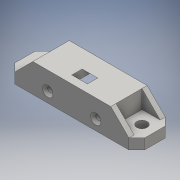
# Autodesk Inventor part: Support_GP2
Saved by Autodesk Inventor 2016 (Build 200138000, 138)
## iProperties
Created: 2016-09-29
Part Number: Support_GP2
Material: Générique
Document SubType Name: Modeling
Designer: LogOut
Density: 1 g/cm^3
Appearance: Par défaut
Author: LogOut
Autodesk Inventor part; units mm, degrees
ref_plane "YZ Plane" through (0, 0, 0) normal (1, 0, 0) x (0, 1, 0)
ref_plane "XZ Plane" through (0, 0, 0) normal (0, 1, 0) x (-1, 0, 0)
sketch "Esquisse1" plane through (0, 0, 0) normal (0, 0, 1) x (1, 0, 0)
  line L0 (-50, 14) -> (50, 14)
  line L1 (50, 14) -> (50, -14)
  line L2 (50, -14) -> (-50, -14)
  line L3 (-50, -14) -> (-50, 14)
  point P0 (0, 0)
  dimension "d0" = 100
  dimension "d1" = 28
  dimension "d2" = 14
  dimension "d3" = 50
  constraints: 8 end point, 2 parallel, 1 horizontal, 1 perpendicular
  measures "d0" distance of L0.start L0.end
  measures "d1" distance of L2.end L0.start
  measures "d2" distance from line of point (0, 0) L0
  measures "d3" distance from line of point (0, 0) L1
extrude "Extrusion1" add sketch "Esquisse1" along normal blind 28
sketch "Esquisse2" plane through (-50, 14, 0) normal (0, 1, 0) x (1, 0, 0)
  line L0 (26, -22) -> (74, -22)
  line L1 (74, -22) -> (74, -6)
  line L2 (74, -6) -> (26, -6)
  line L3 (26, -6) -> (26, -22)
  line L4 (0, 0) -> (100, 0) projected
  line L5 (0, 0) -> (0, -28) projected
  line L6 (100, -28) -> (0, -28) projected
  line L7 (100, 0) -> (100, -28) projected
  point P0 (50, 0)
  dimension "d6" = 26
  dimension "d7" = 48
  dimension "d8" = 26
  dimension "d9" = 6
  dimension "d10" = 6
  dimension "d11" = 16
  constraints: 8 end point, 2 parallel, 1 horizontal, 1 perpendicular
  measures "d6" distance between parallel lines of L5 L3
  measures "d7" distance between parallel lines of L1 L3
  measures "d8" distance between parallel lines of L7 L1
  measures "d9" distance between parallel lines of L4 L2
  measures "d10" distance between parallel lines of L6 L0
  measures "d11" distance of L2.end L0.start
extrude "Extrusion2" cut sketch "Esquisse2" against normal blind 24 contours L3 L2 L1 L0
ref_plane "Plan de construction1" through (-24, 14, 14) normal (0, 0, 1) x (1, 0, 0)
sketch "Esquisse3" plane through (-24, 14, 14) normal (0, 0, 1) x (1, 0, 0)
  line L0 (110.7171, 2) -> (-26, 2)
  line L1 (70, 2) -> (54, -18)
  line L2 (-6, -18) -> (-26, 2)
  line L3 (-26, 2) -> (-81.3521, 2)
  line L4 (74, -28) -> (-26, -28) projected
  line L5 (110.7171, 2) -> (110.7171, -53.3012)
  line L6 (110.7171, -53.3012) -> (-81.3521, -53.3012)
  line L7 (-81.3521, -53.3012) -> (-81.3521, 2)
  line L8 (-6, 2) -> (-6, -28)
  line L9 (-26, -28) -> (74, -28) projected
  line L10 (-6, -28) -> (54, -28)
  line L11 (54, -53.3012) -> (54, 2)
  point P0 (24, -14)
  point P1 (54.2399, -28)
  point P2 (-6.2399, -28)
  dimension "d25" = 60
  dimension "d26" = 30
  dimension "d27" = 30
  constraints: 20 end point, 10 point on line, 5 perpendicular, 1 collinear, 1 horizontal, 1 vertical
  measures "d25" distance between parallel lines of L11 L8
  measures "d26" distance from line of point (24, -14) L11
  measures "d27" distance from line of point (24, -14) L8
extrude "Extrusion3" cut sketch "Esquisse3" along normal blind 14 and the other way blind 3 contours L5 L6 L11 L1 L0 | L1 L11 L0 | L6 L7 L3 L2 L8 L4 L11 | L8 L2 L0
sketch "Esquisse7" plane through (-50, -10, 0) normal (0, 1, 0) x (1, 0, 0)
  line L0 (68.5, -14) -> (31.5, -14)
  line L1 (74, -6) -> (74, -22) projected
  line L2 (26, -6) -> (74, -6) projected
  point P0 (50, 0)
  dimension "d61" = 37
  dimension "d62" = 5.5
  dimension "d63" = 8
  constraints: 2 end point, 1 horizontal
  measures "d61" distance of L0.start L0.end
  measures "d62" distance from line of L1 L0.start
  measures "d63" distance between parallel lines of L0 L2
hole "Perçage2" at (18.5, -10, 14) at (-18.5, -10, 14) direction (0, -1, 0) diameter 4 end through all
chamfer "Chanfrein1" distance 2 angle 45 6 edges at (-18.5, -14, 12) (18.5, -14, 12) (24, 14, 14) (0, 14, 22) (-24, 14, 14) (0, 14, 6)
sketch "Esquisse8" plane through (0, 0, 28) normal (0, 0, 1) x (1, 0, 0)
  line L0 (6, -8) -> (-6, -8)
  line L1 (-6, -8) -> (-6, 0)
  line L2 (-6, 0) -> (6, 0)
  line L3 (6, 0) -> (6, -8)
  line L4 (-30, -14) -> (30, -14) projected
  point P0 (0, 0)
  point P1 (-28, -14)
  point P2 (28, -14)
  dimension "d74" = 12
  dimension "d75" = 8
  dimension "d76" = 6
  dimension "d77" = 6
  constraints: 8 end point, 2 parallel, 1 horizontal, 1 perpendicular
  measures "d74" distance of L0.start L0.end
  measures "d75" distance between parallel lines of L0 L2
  measures "d76" distance between parallel lines of L4 L0
  measures "d77" distance from line of point (0, 0) L3
extrude "Extrusion6" cut sketch "Esquisse8" against normal blind 6
chamfer "Chanfrein2" distance 8 distance2 6 1 edges at (0, 0, 22) measured on face at (2, 8, 22)
sketch "Esquisse10" plane through (-50, 14, 11) normal (0, 1, 0) x (1, 0, 0)
  line L0 (26, 5) -> (74, 5) projected
  line L1 (0, 11) -> (0, 0) projected
  line L2 (100, 11) -> (100, 0) projected
  line L3 (108, 0) -> (100, 0) projected
  line L4 (100, 0) -> (100, 29.3143)
  line L5 (100, 29.3143) -> (0, 29.3143)
  line L6 (0, 4) -> (0, 0) projected
  line L7 (0, 29.3143) -> (0, 0)
  line L8 (0, 5) -> (100, 5)
  point P0 (50, 11)
  point P1 (104, 4)
  point P2 (0, -10)
  point P3 (83.4286, 5)
  constraints: 8 end point, 3 collinear, 2 point on line, 1 perpendicular, 1 vertical, 1 other
extrude "Extrusion8" cut sketch "Esquisse10" against normal through all
move faces "Déplacer2" translate (0, 0, 3) faces at (36.6667, 4.6667, 11) (-43.3333, 4.6667, 11)
chamfer "Chanfrein3" distance 14 angle 45 2 edges at (30, 0, 14) (-30, 0, 14)
sketch "Esquisse11" plane through (0, 0, 28) normal (0, 0, 1) x (1, 0, 0)
  line L0 (30, -10) -> (44, -10)
  line L1 (44, -10) -> (44, 10)
  line L2 (44, 10) -> (30, 10)
  line L3 (30, 10) -> (30, -10)
  line L4 (0, 23.1019) -> (0, 45.1351)
  line L5 (30, -14) -> (30, 14) projected
  line L6 (44, -14) -> (44, 14) projected
  line L7 (30, -14) -> (44, -14) projected
  line L8 (44, 14) -> (30, 14) projected
  line L9 (-30, -10) -> (-44, -10)
  line L10 (-44, -10) -> (-44, 10)
  line L11 (-44, 10) -> (-30, 10)
  line L12 (-30, 10) -> (-30, -10)
  line L13 (-30, -14) -> (-30, 14)
  line L14 (-44, -14) -> (-44, 14)
  line L15 (-30, -14) -> (-44, -14)
  line L16 (-44, 14) -> (-30, 14)
  point P0 (0, 0)
  dimension "d100" = 4
  dimension "d101" = 4
  constraints: 26 end point, 8 symmetric about line, 2 collinear, 2 parallel, 1 horizontal, 1 perpendicular, 1 vertical
  measures "d100" distance between parallel lines of L7 L0
  measures "d101" distance between parallel lines of L8 L2
extrude "Extrusion9" cut sketch "Esquisse11" against normal blind 14 contours L3 L2 L1 L0 | L9 L10 L11 L12
chamfer "Chanfrein4" distance 6 angle 45 4 edges at (50, 14, 10) (50, -14, 10) (-50, 14, 10) (-50, -14, 10)
sketch "Esquisse12" plane through (30, 10, 14) normal (0, 0, 1) x (1, 0, 0)
  line L0 (10, -10) -> (-70, -10)
  line L1 (20, -2) -> (20, -18) projected
  line L2 (-80, -18) -> (-80, -2) projected
  point P0 (-30, -10)
  dimension "d107" = 10
  dimension "d108" = 10
  constraints: 2 end point, 1 horizontal
  measures "d107" distance from line of L1 L0.start
  measures "d108" distance from line of L2 L0.end
hole "Perçage3" at (40, 0, 14) at (-40, 0, 14) direction (0, 0, -1) diameter 8 end through all
